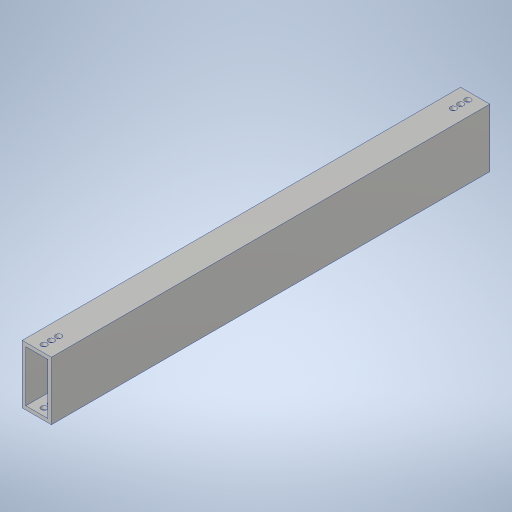
# Autodesk Inventor part: Cl1-003
Saved by Autodesk Inventor 2023.4 (Build 274418000, 418)
## iProperties
Created: 2025-01-18
Part Number: Cl1-003
Material: Aluminum 6061
Document SubType Name: Modeling
Designer: mavericks
Mass: 304.185 g
Surface Area: 718.547 cm^2
Volume: 112.661 cm^3
Density: 2.7 g/cm^3
Appearance: Aluminum - Flat
RuleStatus: InUse
AfterDocNew0: SHOW
AfterDocOpen0: SHOW
Author: mavericks
Autodesk Inventor part; units mm, degrees
ref_plane "YZ Plane" through (0, 0, 0) normal (1, 0, 0) x (0, 1, 0)
ref_plane "XZ Plane" through (0, 0, 0) normal (0, 1, 0) x (-1, 0, 0)
ref_plane "XY Plane" through (0, 0, 0) normal (0, 0, 1) x (1, 0, 0)
sketch "Sketch1" plane through (0, 0, 0) normal (0, 0, 1) x (1, 0, 0)
  line L0 (-12.7, -25.4) -> (12.7, -25.4)
  line L1 (12.7, -25.4) -> (12.7, 25.4)
  line L2 (12.7, 25.4) -> (-12.7, 25.4)
  line L3 (-12.7, 25.4) -> (-12.7, -25.4)
  line L4 (-12.7, -25.4) -> (12.7, 25.4) construction
  line L5 (12.7, -25.4) -> (-12.7, 25.4) construction
  line L6 (-9.525, 22.225) -> (9.525, 22.225)
  line L7 (9.525, 22.225) -> (9.525, -22.225)
  line L8 (9.525, -22.225) -> (-9.525, -22.225)
  line L9 (-9.525, -22.225) -> (-9.525, 22.225)
  point P0 (0, 0)
  dimension "width" = 25.4
  dimension "height" = 50.8
  dimension "thickness" = 3.175
  constraints: 20 end point, 4 parallel, 2 midpoint, 2 perpendicular, 1 horizontal, 3 other
  measures "width" distance of L2.end L1.end
  measures "height" distance of L1.end L0.end
  measures "thickness" distance between parallel lines of L2 L6
extrude "Extrusion1" add sketch "Sketch1" along normal mid plane 381
sketch "Sketch2" plane through (-12.7, 25.4, 190.5) normal (0, 1, 0) x (1, 0, 0)
  line L0 (0, 381) -> (25.4, 381) projected
  line L1 (25.4, 381) -> (25.4, 0) projected
  line L2 (25.4, 0) -> (0, 0) projected
  point P0 (12.7, 190.5)
  point P1 (12.7, 374.65)
  point P2 (12.7, 368.3)
  point P3 (12.7, 361.95)
  point P4 (12.7, 6.35)
  point P5 (12.7, 12.7)
  point P6 (12.7, 19.05)
  point P7 (12.7, 0)
  dimension "d5" = 6.35
  dimension "d6" = 6.35
  dimension "d7" = 6.35
  dimension "d8" = 12.7
  dimension "d16" = 12.7
  dimension "d17" = 6.35
  dimension "d18" = 6.35
  dimension "d19" = 6.35
  constraints: 4 vertical alignment, 1 midpoint
  measures "d5" distance from line of L0 point (12.7, 374.65)
  measures "d6" distance of point (12.7, 368.3) point (12.7, 374.65)
  measures "d7" distance of point (12.7, 368.3) point (12.7, 361.95)
  measures "d8" distance from line of L1 point (12.7, 374.65)
  measures "d16" distance from line of L1 point (12.7, 6.35)
  measures "d17" distance of point (12.7, 0) point (12.7, 6.35)
  measures "d18" distance of point (12.7, 6.35) point (12.7, 12.7)
  measures "d19" distance of point (12.7, 12.7) point (12.7, 19.05)
hole "Hole1" at (0, 25.4, -184.15) at (0, 25.4, -177.8) at (0, 25.4, -171.45) at (0, 25.4, 171.45) at (0, 25.4, 177.8) at (0, 25.4, 184.15) direction (0, -1, 0) diameter 5.1054 end through all clearance for "Flat Head Machine Screw (82)" size "#10" standard "Ansi Unified Screw Threads"
equation "\"d6\" = d5"
equation "\"d7\" = d6"
equation "\"d18\" = d17"
equation "\"d19\" = d18"
body "Solid1"
